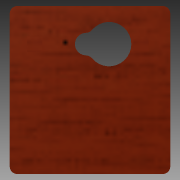
# Autodesk Inventor part: wall-middle
Saved by Autodesk Inventor 2015 (Build 190159000, 159)
## iProperties
Created: 2014-07-16
Part Number: wall-middle
Material: Wood (Oak)
Document SubType Name: Modeling
Designer: pc
Density: 0.76 g/cm^3
Appearance: White Oak - Natural Medium Gloss
Author: pc
Autodesk Inventor part; units mm, degrees
ref_plane "YZ Plane" through (0, 0, 0) normal (1, 0, 0) x (0, 1, 0)
ref_plane "XZ Plane" through (0, 0, 0) normal (0, 1, 0) x (-1, 0, 0)
ref_plane "XY Plane" through (0, 0, 0) normal (0, 0, 1) x (1, 0, 0)
sketch "Sketch1" plane through (0, 0, 0) normal (0, 1, 0) x (-1, 0, 0)
  line L0 (-21, 22) -> (21, 22)
  line L1 (21, 22) -> (21, -22)
  line L2 (21, -22) -> (-21, -22)
  line L3 (-21, -22) -> (-21, 22)
  line L4 (-21, 22) -> (21, -22) construction
  line L5 (21, 22) -> (-21, -22) construction
  point P0 (0, 0)
  dimension "d0" = 42
  dimension "d1" = 44
  constraints: 12 end point, 2 midpoint, 2 parallel, 1 horizontal, 1 perpendicular
  measures "d0" distance of L1.end L2.end
  measures "d1" distance of L0.end L1.end
extrude "wall2" add sketch "Sketch1" along normal blind 6.4
sketch "Sketch7" plane through (0, 6.4, 0) normal (0, 1, 0) x (1, 0, 0)
  line L0 (5, -22) -> (5, 22) construction
  line L1 (21, 22) -> (-21, 22) projected
  line L2 (-21, -22) -> (21, -22) projected
  line L3 (-21, 12) -> (21, 12) construction
  line L4 (21, -22) -> (21, 22) projected
  line L5 (-21, 22) -> (-21, -22) projected
  circle A0 centre (5, 12) radius 5.81
  point P0 (0, 0)
  dimension "d74" = 34
  dimension "d75" = 26
  dimension "d76" = 11.62
  constraints: 6 point on line, 4 end point, 1 centre point, 1 horizontal, 1 vertical
  measures "d74" distance between parallel lines of L2 L3
  measures "d75" distance between parallel lines of L5 L0
  measures "d76" diameter of A0
extrude "bigcircle" cut sketch "Sketch7" against normal blind 6.4 contours A0
sketch "Sketch8" plane through (0, 6.4, 0) normal (0, 1, 0) x (1, 0, 0)
  line L0 (-21, -22) -> (-21, 22) projected
  line L1 (-21, 12) -> (21, 12) construction
  line L2 (21, 22) -> (21, -22) projected
  line L3 (5, 22) -> (5, -22) construction
  line L4 (21, -22) -> (21, 22) projected
  line L5 (21, 22) -> (-21, 22) projected
  line L6 (-21, -22) -> (21, -22) projected
  circle A0 centre (-1, 12) radius 2.96
  point P0 (0, 0)
  dimension "d81" = 26
  dimension "d82" = 34
  dimension "d83" = 5.92
  dimension "d84" = 6
  constraints: 5 point on line, 4 end point, 1 centre point, 1 perpendicular, 1 vertical
  measures "d81" distance between parallel lines of L0 L3
  measures "d82" distance between parallel lines of L6 L1
  measures "d83" diameter of A0
  measures "d84" distance from line of A0.centre L3
extrude "smallcircle" cut sketch "Sketch8" against normal blind 6.4 contours A0
fillet "Fillet4" radius 2 1 edges at (-0.0829, 3.2, -14.8143)
fillet "Fillet5" radius 2 1 edges at (-0.0829, 3.2, -9.1857)
fillet "Fillet6" radius 2 1 edges at (-21, 3.2, -22)
fillet "Fillet7" radius 2 1 edges at (21, 3.2, -22)
fillet "Fillet8" radius 2 1 edges at (-21, 3.2, 22)
fillet "Fillet9" radius 2 1 edges at (21, 3.2, 22)
sketch "Sketch9" plane through (0, 6.4, 0) normal (0, 1, 0) x (1, 0, 0)
  line L0 (11.31, 17.1525) -> (11.31, -6.1616) construction
  line L1 (10.81, 14.2171) -> (10.81, 9.0836) construction
  arc A0 (0.512, 8.3102) -> (0.512, 15.6898) centre (5, 12) ccw projected
  line L2 (-21, 12) -> (18.6779, 12) construction
  line L3 (11.31, 10) -> (15.31, 10)
  line L4 (15.31, 10) -> (15.31, 14)
  line L5 (15.31, 14) -> (11.31, 14)
  line L6 (11.31, 14) -> (11.31, 10)
  line L7 (11.31, 10) -> (15.31, 14) construction
  line L8 (15.31, 10) -> (11.31, 14) construction
  line L9 (-21, 20) -> (-21, -20) projected
  line L10 (-16.49, 14) -> (-12.49, 14)
  line L11 (-12.49, 14) -> (-12.49, 10)
  line L12 (-12.49, 10) -> (-16.49, 10)
  line L13 (-16.49, 10) -> (-16.49, 14)
  line L14 (-16.49, 14) -> (-12.49, 10) construction
  line L15 (-12.49, 14) -> (-16.49, 10) construction
  point P0 (0, 0)
  point P1 (13.31, 12)
  point P2 (-14.49, 12)
  dimension "d93" = 0.5
  dimension "d94" = 4
  dimension "d95" = 23.3
  constraints: 30 end point, 5 perpendicular, 4 midpoint, 4 parallel, 4 point on line, 3 horizontal, 2 vertical, 1 collinear, 1 tangent
  measures "d93" distance between parallel lines of L0 L1
  measures "d94" distance of L3.start L3.end
  measures "d95" distance between parallel lines of L1 L11
extrude "Extrusion7" add sketch "Sketch9" along normal blind 4
equation "\"d0\" = wallw"
equation "\"d1\" = wallh"
equation "\"d72\" = wall2_thick"
equation "\"d74\" = distancefrombottom"
equation "\"d75\" = distancefromleft"
equation "\"d76\" = servobigcircledia"
equation "\"d79\" = wall2_thick"
equation "\"d81\" = distancefromleft"
equation "\"d82\" = distancefrombottom"
equation "\"d83\" = servosmallcircledia"
equation "\"d85\" = wall2_thick"
equation "\"d89\" = cornerrad"
equation "\"d90\" = cornerrad"
equation "\"d91\" = cornerrad"
equation "\"d92\" = cornerrad"
equation "\"d94\" = servomountsquare"
equation "\"d96\" = servomounth"
equation "\"printer3dtolerance\" = 0.12"
equation "\"wallw\" = 42"
equation "\"wallh\" = 44"
equation "\"cornerrad\" = 2"
equation "\"baseextra\" = 2"
equation "\"wall1_thick\" = 8"
equation "\"wall2_thick\" = 6.4"
equation "\"wall3_thick\" = 4"
equation "\"wall1slot\" = 8.12"
equation "\"wall2slot\" = 6.52"
equation "\"wall3slot\" = 4.12"
equation "\"gap2\" = 28"
equation "\"baseh\" = 79.12"
equation "\"basew\" = 44"
equation "\"base_thick\" = 6"
equation "\"base_slots_depth\" = 4"
equation "\"servomounth\" = 4"
equation "\"servosmallcircledia\" = 5.92"
equation "\"servomountsquare\" = 4"
equation "\"servobigcircledia\" = 11.62"
equation "\"servo9gw\" = 22.8"
equation "\"distancefromleft\" = 26"
equation "\"servopolygonl\" = 5.92"
equation "\"servopolygonr\" = 6.12"
equation "\"distancefrombottom\" = 34"
equation "\"d49\" = distancefrombottom"
equation "\"adapterh\" = 16"
equation "\"wall3slotd\" = 2"
equation "\"adapterw\" = 32"
equation "\"wall3slotd_1\" = 2"
equation "\"wall3slotw\" = 36"
equation "\"armslotd\" = 2"
equation "\"armthick\" = 3"
equation "\"armw\" = 36"
equation "\"fanhb\" = 11"
equation "\"fanhs\" = 9.6"
equation "\"adapterwallthick\" = 6"
equation "\"adapterwallslotd\" = 2"
equation "\"armhornthick\" = 3"
equation "\"hornscrewholed\" = 2"
equation "\"hornscrewheadd\" = 3"
equation "\"hornthick\" = 1.5"
body "Solid2"
